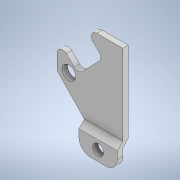
# Autodesk Inventor part: PartE_2
Saved by Autodesk Inventor 2020 (Build 240168000, 168)
## iProperties
Created: 2021-05-26
Part Number: PartE_2
Material: Generic
Document SubType Name: Modeling
Designer: Ed
Density: 1 g/cm^3
Appearance: Default
Author: Ed
Autodesk Inventor part; units mm, degrees
ref_plane "YZ Plane" through (0, 0, 0) normal (1, 0, 0) x (0, 1, 0)
ref_plane "XZ Plane" through (0, 0, 0) normal (0, 1, 0) x (-1, 0, 0)
ref_plane "XY Plane" through (0, 0, 0) normal (0, 0, 1) x (1, 0, 0)
sketch "Sketch1" plane through (0, 0, 0) normal (0, 0, 1) x (1, 0, 0)
  circle A0 centre (0, 0) radius 1.25
  line L0 (-4.75, 9.95) -> (2.5, 9.95)
  line L1 (2.5, 9.95) -> (2.5, -4.95)
  line L2 (2.5, -4.95) -> (-4.75, -4.95)
  line L3 (-4.75, -4.95) -> (-4.75, 9.95)
  line L4 (-4.75, 4.85) -> (-9.65, 4.85)
  line L5 (-9.65, 4.85) -> (-9.65, 0.15)
  line L6 (-9.65, 0.15) -> (-4.75, 0.15)
  line L7 (-4.75, 0.15) -> (-4.75, 4.85)
  line L8 (-4.75, -4.95) -> (-9.65, 0.15)
  line L9 (-9.65, 4.85) -> (-4.75, 9.95)
  line L10 (-9.65, 4.85) -> (-13.2555, 8.3141)
  line L11 (-4.75, 9.95) -> (-8.2862, 13.4862)
  line L12 (-13.2555, 8.3141) -> (-8.2862, 13.4862)
  circle A1 centre (-7.5, 1) radius 1.25
  line L13 (-9.5461, 4.9582) -> (-13.1516, 8.4223)
  line L14 (-4.8539, 9.8418) -> (-8.3902, 13.3781)
  line L15 (2.4, 9.95) -> (2.4, -4.95)
  line L16 (-9.65, 0.2541) -> (-4.65, -4.95)
  point P0 (-8.4165, 0.15)
  point P1 (-6.5835, 0.15)
  point P2 (-9.55, 0.15)
  point P3 (-4.75, -4.8459)
  dimension "d26" = 4.95
  dimension "d27" = 7.25
  dimension "d28" = 2.5
  dimension "d29" = 4.9
  dimension "d30" = 14.9
  dimension "d31" = 5.1
  dimension "d32" = 5.1
  dimension "d33" = 90
  dimension "d34" = 135
  dimension "d36" = 0
  dimension "d37" = 0
  dimension "d38" = 2.5
  dimension "d39" = 5
  dimension "d40" = 2.5
  dimension "d41" = 1
  dimension "d42" = 7.5
  dimension "d43" = 0.15
  dimension "d44" = 0.15
  dimension "d54" = 0.1
  dimension "d55" = 0.1
  constraints: 34 end point, 9 point on line, 8 parallel, 3 perpendicular, 2 centre point, 2 horizontal
  measures "d26" distance from line of A0.centre L2
  measures "d27" distance of L1.end L3.start
  measures "d28" distance from line of A0.centre L1
  measures "d29" distance between parallel lines of L3 L5
  measures "d30" distance of L3.start L0.start
  measures "d31" distance from line of L3.start L6
  measures "d32" distance from line of L0.start L4
  measures "d33" angle of L10 L9
  measures "d34" angle of L0 L11
  measures "d36" distance of point (0, 0) A0.centre
  measures "d37" distance of point (0, 0) A0.centre
  measures "d38" diameter of A0
  measures "d39" distance between parallel lines of L12 L9
  measures "d40" diameter of A1
  measures "d41" vertical distance of A1.centre point (0, 0)
  measures "d42" horizontal distance of A1.centre point (0, 0)
  measures "d43" distance between parallel lines of L13 L10
  measures "d44" distance between parallel lines of L11 L14
  measures "d54" distance of L16.end L3.start
  measures "d55" distance between parallel lines of L1 L15
extrude "Extrusion1" add sketch "Sketch1" along normal blind 1 contours A0 | L0 L15 L2 L16 L3 | L3 L4 L9 | L3 L6 A1 L16 L5 L4 | L3 L16 L6 A1
sketch "Sketch7" plane through (0, 0, 0) normal (0, 0, -1) x (-1, 0, 0)
  line L0 (4.65, -4.95) -> (-2.4, -4.95) projected
  line L1 (9.65, 0.2541) -> (4.65, -4.95) projected
  line L2 (9.65, 4.85) -> (9.65, 0.2541) projected
  line L3 (4.75, 9.95) -> (9.65, 4.85) projected
  line L4 (-2.4, 9.95) -> (4.75, 9.95) projected
  line L5 (-2.4, -4.95) -> (-2.4, 9.95) projected
  circle A0 centre (7.5, 1) radius 1.25 projected
  line L6 (4.65, -4.95) -> (-2.4, -4.95) projected
  line L7 (-2.4, -4.95) -> (4.65, -4.95)
  line L8 (4.65, -4.95) -> (4.65, -9.45)
  line L9 (4.65, -9.45) -> (-2.4, -9.45)
  line L10 (-2.4, -9.45) -> (-2.4, -4.95)
  circle A1 centre (1.125, -7.55) radius 1
  line L11 (4.75, 9.95) -> (8.2855, 13.4855)
  line L12 (4.75, 9.95) -> (9.75, 9.95) construction
  line L13 (9.65, 4.85) -> (13.1855, 8.3855)
  line L14 (9.65, 4.85) -> (14.65, 4.85) construction
  line L15 (13.1855, 8.3855) -> (8.2855, 13.4855)
  line L16 (9.5114, 4.9942) -> (13.0469, 8.5298)
  line L17 (-2.4, -4.95) -> (-2.4, 9.95) projected
  line L18 (-2.4, 9.85) -> (4.8461, 9.85)
  line L19 (4.8461, 9.85) -> (8.3816, 13.3855)
  point P0 (0, 0)
  dimension "d56" = 0
  dimension "d57" = 4.5
  dimension "d58" = 2
  dimension "d59" = 3.525
  dimension "d60" = 2.6
  dimension "d63" = 5
  dimension "d64" = 45
  dimension "d65" = 5
  dimension "d66" = 45
  dimension "d68" = 0.2
  dimension "d69" = 0.1
  constraints: 24 end point, 5 parallel, 5 point on line, 3 horizontal, 2 equal length, 1 centre point, 1 perpendicular
  measures "d56" distance from line of L0.start L8
  measures "d57" distance between parallel lines of L0 L9
  measures "d58" diameter of A1
  measures "d59" distance from line of L10 A1.centre
  measures "d60" distance from line of L0 A1.centre
  measures "d63" distance of L3.start L11.end
  measures "d64" angle of L12 L11
  measures "d65" distance of L2.start L13.end
  measures "d66" angle of L14 L13
  measures "d68" distance between parallel lines of L13 L16
  measures "d69" distance between parallel lines of L4 L18
extrude "Extrusion5" add sketch "Sketch7" against normal mid plane 2 contours L8 L9 L10 L0 | L19 L15 L16 L3
fillet "Fillet2" radius 2.1 2 edges at (-4.65, -9.45, 0) (2.4, -9.45, 0)
sketch "Sketch8" plane through (0, 0, 1) normal (0, 0, 1) x (1, 0, 0)
  line L0 (2.4, 9.95) -> (-4.75, 9.95) projected
  line L1 (-4.75, 9.95) -> (-4.8461, 9.85) projected
  line L2 (2.4, -7.35) -> (2.4, 9.95) projected
  line L3 (-4.75, 9.95) -> (-4.8461, 9.85) projected
  line L4 (-4.8461, 9.85) -> (2.4, 9.85)
  point P0 (0, 0)
  constraints: 2 end point, 1 perpendicular, 1 point on line
extrude "Extrusion6" cut sketch "Sketch8" against normal up to surface (1 mm away)
chamfer "Chamfer1" distance 1 angle 45 2 edges at (-1.125, -4.95, -1) (-7.1787, 7.4221, -1)
sketch "Sketch9" plane through (0, 0, 1) normal (0, 0, 1) x (1, 0, 0)
  line L0 (-4.65, -4.95) -> (2.4, -4.95) projected
  line L1 (2.4, -5.95) -> (-4.65, -5.95) projected
  line L2 (2.4, 9.85) -> (-4.8461, 9.85) projected
  line L3 (-4.8461, 9.85) -> (-8.3816, 13.3855) projected
  line L4 (-8.3816, 13.3855) -> (-13.0469, 8.5298) projected
  line L5 (-13.0469, 8.5298) -> (-9.5114, 4.9942) projected
  line L6 (-9.5114, 4.9942) -> (-9.65, 4.85) projected
  line L7 (-9.65, 4.85) -> (-9.65, 0.2541) projected
  line L8 (-9.65, 0.2541) -> (-4.65, -4.95) projected
  line L9 (-4.65, -4.95) -> (-4.65, -7.35) projected
  arc A0 (-4.65, -7.35) -> (-2.55, -9.45) centre (-2.55, -7.35) ccw projected
  line L10 (-2.55, -9.45) -> (0.3, -9.45) projected
  arc A1 (0.3, -9.45) -> (2.4, -7.35) centre (0.3, -7.35) ccw projected
  line L11 (2.4, -7.35) -> (2.4, 9.85) projected
  circle A2 centre (-1.125, -7.55) radius 1 projected
  circle A3 centre (-7.5, 1) radius 1.25 projected
  point P0 (0, 0)
extrude "Extrusion7" cut sketch "Sketch9" against normal blind 1 contours L1 L11 A1 L10 A0 L9
chamfer "Chamfer2" distance 1 angle 45 1 edges at (-1.125, -5.95, 1)
sketch "Sketch10" plane through (0, 0, 0) normal (0, 0, 1) x (1, 0, 0)
  circle A0 centre (-1.125, -7.55) radius 1 projected
  circle A1 centre (-1.125, -7.55) radius 1.9
  point P0 (0, 0)
  dimension "d80" = 3.8
  constraints: 1 centre point, 1 coincident
  measures "d80" diameter of A1
extrude "Extrusion8" cut sketch "Sketch10" along normal up to surface (1 mm away)
sketch "Sketch11" plane through (0, 0, 1) normal (0, 0, 1) x (1, 0, 0)
  line L0 (-6.2966, 11.2255) -> (-10.8, 6.5383)
  line L1 (-10.8, 6.5383) -> (-5.7523, 1.6886)
  line L2 (-5.7523, 1.6886) -> (-1.2489, 6.3757)
  line L3 (-1.2489, 6.3757) -> (-6.2966, 11.2255)
  line L4 (-6.2966, 11.2255) -> (-5.7523, 1.6886) construction
  line L5 (-10.8, 6.5383) -> (-1.2489, 6.3757) construction
  line L6 (-8.3816, 13.3855) -> (-13.0469, 8.5298) projected
  line L7 (-13.0469, 8.5298) -> (-9.5114, 4.9942) projected
  line L8 (-4.8461, 9.85) -> (-8.3816, 13.3855) projected
  line L9 (-4.8461, 9.85) -> (2.4, 9.85) projected
  line L10 (-4.8461, 9.85) -> (-4.8551, 9.8406)
  line L11 (-4.8461, 9.85) -> (-9.5114, 4.9942) projected
  point P0 (0, 0)
  point P1 (-6.0245, 6.457)
  point P2 (-10.9252, 6.408)
  point P3 (-6.2599, 11.2638)
  point P4 (-9.3585, 5.1534)
  dimension "d83" = 7
  dimension "d85" = 6.5
  dimension "d86" = 3.5
  dimension "d89" = 6.5
  constraints: 14 end point, 3 parallel, 2 midpoint, 2 point on line, 1 perpendicular
  measures "d83" distance of L2.end L0.start
  measures "d85" distance from line of L6 point (-6.024, 6.457)
  measures "d86" distance from line of point (-6.024, 6.457) L7
  measures "d89" distance between parallel lines of L1 L3
extrude "Extrusion9" cut sketch "Sketch11" against normal up to surface (2 mm away)
fillet "Fillet3" radius 1 1 edges at (-5.7523, 1.6886, 0.5)
fillet "Fillet4" radius 1 5 edges at (-9.3585, 5.1534, 0.5) (-9.65, 4.85, 0.5) (-1.2489, 6.3757, 0.5) (-4.8551, 9.8406, 0.5) (-4.8461, 9.85, 0.5)
mirror "Mirror2" about plane through (-3.625, 2.5, 1) normal (0, 0, 1) remove original yes
body "Solid1"
